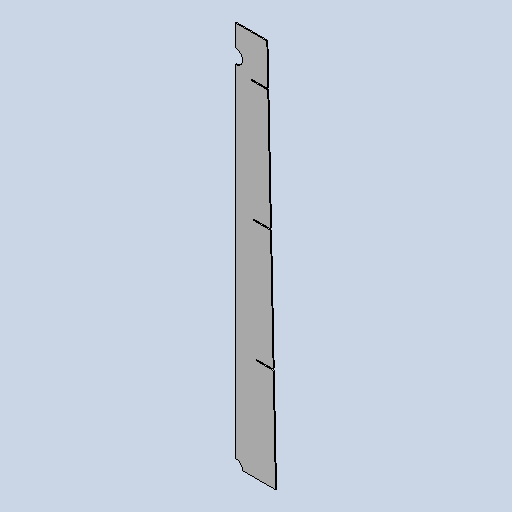
# Autodesk Inventor part: GBK 3212 central second rib
Saved by Autodesk Inventor 2026.2 (Build 302298010, 298A)
## iProperties
Created: 2026-04-17
Part Number: GBK 3212 central second rib
Material: Steel
Document SubType Name: Sheet Metal
Designer: pokla
Mass: 7201.32 g
Surface Area: 4740.76 cm^2
Volume: 917.366 cm^3
Density: 7.85 g/cm^3
Flat Pattern Width: 16.6667 cm
Flat Pattern Length: 159.962 cm
Flat Pattern Area: 2666.04 cm^2
Sheet Metal Rule: Default
Sheet Metal Width: 166,667 mm
Sheet Metal Length: 1599,625 mm
Sheet Metal Area: 266604,096 mm^2
Appearance: Default
Author: admin
Autodesk Inventor part; units mm, degrees
ref_plane "YZ Plane" through (0, 0, 0) normal (1, 0, 0) x (0, 1, 0)
ref_plane "XZ Plane" through (0, 0, 0) normal (0, 1, 0) x (-1, 0, 0)
ref_plane "XY Plane" through (0, 0, 0) normal (0, 0, 1) x (1, 0, 0)
sketch "Sketch1" plane through (0, 0, 0) normal (0, 0, 1) x (1, 0, 0)
  line L0 (0, 0) -> (0, 4438.8737)
  line L1 (0, 4438.8737) -> (100, 4438.8737)
  line L2 (100, 4438.8737) -> (200, 0)
  line L3 (200, 0) -> (0, 0)
  circle A0 centre (0, 0) radius 30
  line L4 (0, 1479.6246) -> (166.6667, 1479.6246)
  line L5 (0, 2959.2492) -> (133.3333, 2959.2492)
  circle A1 centre (0, 1479.6246) radius 30
  circle A2 centre (0, 2959.2492) radius 30
  line L6 (190.8761, 405) -> (120.8761, 405)
  line L7 (120.8761, 405) -> (120.8761, 410)
  line L8 (120.8761, 410) -> (190.8761, 410)
  line L9 (190.8761, 410) -> (190.8761, 405)
  line L10 (109.6148, 909.8732) -> (179.6148, 909.8732)
  line L11 (179.6148, 904.8732) -> (109.6148, 904.8732)
  line L12 (109.6148, 904.8732) -> (109.6148, 909.8732)
  line L13 (179.6148, 909.8732) -> (179.6148, 904.8732)
  line L14 (98.3535, 1409.7463) -> (168.3535, 1409.7463)
  line L15 (168.3535, 1404.7463) -> (98.3535, 1404.7463)
  line L16 (98.3535, 1404.7463) -> (98.3535, 1409.7463)
  line L17 (168.3535, 1409.7463) -> (168.3535, 1404.7463)
  line L18 (87.0923, 1909.6195) -> (157.0923, 1909.6195)
  line L19 (157.0923, 1904.6195) -> (87.0923, 1904.6195)
  line L20 (87.0923, 1904.6195) -> (87.0923, 1909.6195)
  line L21 (157.0923, 1909.6195) -> (157.0923, 1904.6195)
  line L22 (75.831, 2409.4927) -> (145.831, 2409.4927)
  line L23 (145.831, 2404.4927) -> (75.831, 2404.4927)
  line L24 (75.831, 2404.4927) -> (75.831, 2409.4927)
  line L25 (145.831, 2409.4927) -> (145.831, 2404.4927)
  line L26 (64.5698, 2909.3658) -> (134.5698, 2909.3658)
  line L27 (134.5698, 2904.3658) -> (64.5698, 2904.3658)
  line L28 (64.5698, 2904.3658) -> (64.5698, 2909.3658)
  line L29 (134.5698, 2909.3658) -> (134.5698, 2904.3658)
  line L30 (53.3085, 3409.239) -> (123.3085, 3409.239)
  line L31 (123.3085, 3404.239) -> (53.3085, 3404.239)
  line L32 (53.3085, 3404.239) -> (53.3085, 3409.239)
  line L33 (123.3085, 3409.239) -> (123.3085, 3404.239)
  line L34 (42.0472, 3909.1122) -> (112.0472, 3909.1122)
  line L35 (112.0472, 3904.1122) -> (42.0472, 3904.1122)
  line L36 (42.0472, 3904.1122) -> (42.0472, 3909.1122)
  line L37 (112.0472, 3909.1122) -> (112.0472, 3904.1122)
  line L38 (0, 1629.6246) -> (163.2874, 1629.6246)
  line L39 (0, 3079.2492) -> (130.6299, 3079.2492)
  point P0 (30, 2959.2492)
  point P1 (0, 2929.2492)
  point P2 (0, 1509.6246)
  point P3 (0, 1449.6246)
  point P4 (0, 30)
  point P5 (30, 0)
  point P6 (190.7634, 410)
  point P7 (179.5022, 909.8732)
  point P8 (168.3535, 1404.7463)
  point P9 (168.2409, 1409.7463)
  point P10 (30, 1479.6246)
  point P11 (157.0923, 1904.6195)
  point P12 (156.9796, 1909.6195)
  point P13 (145.831, 2404.4927)
  point P14 (145.7184, 2409.4927)
  point P15 (134.5698, 2904.3658)
  point P16 (134.4571, 2909.3658)
  point P17 (0, 2989.2492)
  dimension "d65" = 100
  dimension "d67" = 200
  dimension "d68" = 60
  dimension "d69" = 1480
  dimension "d70" = 1480
  dimension "d71" = 1480
  dimension "d72" = 5
  dimension "d73" = 70
  dimension "d74" = 410
  dimension "d77" = 500
  dimension "d82" = 120
  dimension "d83" = 150
  measures "d65" distance of L0.end L1.end
  measures "d67" distance of L2.end L0.start
  measures "d68" diameter of A0
  measures "d69" distance of L4.end L2.end
  measures "d70" distance of L4.end L5.end
  measures "d71" distance of L1.end L5.end
  measures "d72" distance of L6.end L7.end
  measures "d73" distance of L6.start L6.end
  measures "d74" distance between parallel lines of L3 L8
  measures "d77" distance of L7.end L10.start
  measures "d82" distance between parallel lines of L5 L39
  measures "d83" distance between parallel lines of L38 L4
extrude "Plate3" add sketch "Sketch1" along normal blind 4 contours L39 L2 L5 A2 L0 | L5 L2 L26 L28 L27 L22 L24 L23 L18 L20 L19 L38 L0 A2 | L38 L2 L4 A1 L0
chamfer "Corner Chamfer2" distance 3 angle 45 6 edges at (157.0923, 1904.6195, 2) (156.9796, 1909.6195, 2) (145.831, 2404.4927, 2) (145.7184, 2409.4927, 2) (134.5698, 2904.3658, 2) (134.4571, 2909.3658, 2)
equation "\"BendRadius\" = Thickness"
equation "\"BendReliefWidth\" = Thickness"
equation "\"BendReliefDepth\" = 0.5 * Thickness"
equation "\"CornerReliefSize\" = 4 * Thickness"
equation "\"MinimumRemnant\" = 2 * Thickness"
equation "\"TransitionRadius\" = BendRadius"
equation "\"JacobiRadiusSize\" = BendRadius"
equation "\"GapSize\" = Thickness"
equation "\"Thickness\" = 4"
body "Solid2"
